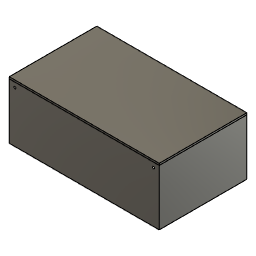
ArduinoLinInterceptor v4 (Autodesk Fusion 360 design; units mm, degrees)
Autodesk Fusion 360 part; units mm, degrees
sketch "Bottom" plane through (0, 0, 0) normal (0, 1, 0) x (1, 0, 0)
  line L0 (0, 0) -> (122, 0)
  line L1 (0, 0) -> (0, -70)
  line L2 (0, -70) -> (122, -70)
  line L3 (122, -70) -> (122, 0)
  line L4 (6, -70) -> (6, 0)
  line L5 (6, -17.75) -> (21.25, -17.75)
  line L6 (6, -66) -> (20, -66)
  line L7 (21.25, -17.75) -> (96.25, -17.75)
  line L8 (20, -66) -> (102.7, -66)
  circle A0 centre (21.25, -17.75) radius 2.5
  circle A1 centre (96.25, -17.75) radius 2.5
  circle A2 centre (20, -66) radius 2.5
  circle A3 centre (102.7, -66) radius 2.5
  point P0 (21.25, -17.75)
  point P1 (20, -66)
  dimension "d3" = 122
  dimension "d4" = 70
  dimension "d10" = 6
  dimension "d11" = 15.25
  dimension "d12" = 14
  dimension "d13" = 75
  dimension "d14" = 82.7
  dimension "d16" = 48.25
  dimension "d17" = 4
  dimension "d33" = 5
  dimension "d34" = 5
  dimension "d35" = 5
  dimension "d36" = 5
  constraint coincident L0.start L1.start
  constraint horizontal L0
  constraint perpendicular L0 L1
  constraint perpendicular L1 L2
  constraint perpendicular L2 L3
  constraint coincident L2 L4.start
  constraint coincident L0 L4.end
  constraint perpendicular L0 L4
  constraint coincident L4 L5.start
  constraint perpendicular L4 L5
  constraint coincident L4 L6.start
  constraint perpendicular L4 L6
  constraint parallel L5 L7
  constraint parallel L6 L8
  constraint coincident P0 L5.end
  constraint coincident P1 L6.end
  constraint coincident L7.end A1.centre
  constraint coincident L8.end A3.centre
  measures "d3" distance of L0.start L0.end
  measures "d4" distance of L0.start L1.end
  measures "d10" distance of L1 L4
  measures "d11" distance of L5.start P0
  measures "d12" distance of L6.start P1
  measures "d13" distance of P0 L7.end
  measures "d14" distance of P1 L8.end
  measures "d16" distance of L5 L6
  measures "d17" distance of L2 L8
  measures "d33" diameter of A0
  measures "d34" diameter of A1
  measures "d35" diameter of A2 L1
  measures "d36" diameter of A3
extrude "Extrude1" add sketch "Bottom" against normal blind 1.5 contours L0 L1 L2 L4 | L0 L2 L3 L4 | L5 L7 A0 | L5 L7 A0 | L6 L8 A2 | L6 L8 A2 | A1 | A3 makes body 1
extrude "Extrude2" add sketch "Bottom" along normal blind 45 and the other way blind 1.5 thin wall 1.5 outside contours L0 L1 L2 L4 | L0 L2 L3 L4 | L5 L7 A0 | L5 L7 A0 | L6 L8 A2 | L6 L8 A2 | A1 | A3 bodies 1
extrude "Extrude3" add sketch "Bottom" along normal blind 3.5 contours L5 L7 A0 | L5 L7 A0 | L6 L8 A2 | L6 L8 A2 | A1 | A3 bodies 1
sketch "ScrewHoles" plane through (0, 3.5, 0) normal (0, 1, 0) x (-1, 0, 0)
  circle A0 centre (-21.25, 17.75) radius 2.5
  circle A1 centre (-21.25, 17.75) radius 2.5
  circle A2 centre (-20, 66) radius 2.5
  line L0 (-21.25, 17.75) -> (-96.25, 17.75)
  circle A3 centre (-102.7, 66) radius 2.5
  line L1 (-122, 70) -> (-122, 0)
  line L2 (-6, 66) -> (-20, 66)
  line L3 (0, 0) -> (-122, 0)
  line L4 (0, 0) -> (0, 70)
  line L5 (0, 70) -> (-122, 70)
  line L6 (-6, 17.75) -> (-21.25, 17.75)
  line L7 (-6, 70) -> (-6, 0)
  line L8 (-20, 66) -> (-102.7, 66)
  circle A4 centre (-96.25, 17.75) radius 2.5
  point P0 (-20, 66)
  point P1 (-21.25, 17.75)
  dimension "d40" = 122
  dimension "d41" = 70
  dimension "d42" = 6
  dimension "d43" = 15.25
  dimension "d44" = 14
  dimension "d45" = 75
  dimension "d46" = 82.7
  dimension "d47" = 48.25
  dimension "d48" = 4
  dimension "d49" = 5
  dimension "d50" = 5
  dimension "d51" = 5
  dimension "d52" = 5
  constraint coincident L3.start L4.start
  constraint perpendicular L3 L4
  constraint perpendicular L4 L5
  constraint perpendicular L1 L5
  constraint coincident L7.start L5
  constraint coincident L7.end L3
  constraint perpendicular L3 L7
  constraint coincident L6.start L7
  constraint perpendicular L6 L7
  constraint coincident L2.start L7
  constraint perpendicular L2 L7
  constraint parallel L0 L6
  constraint parallel L2 L8
  constraint coincident P1 A0.centre
  constraint coincident P0 A2.centre
  constraint coincident L0.end A4.centre
  constraint coincident A3.centre L8.end
  measures "d40" distance of L3.start L1.end
  measures "d41" distance of L4.end L3.start
  measures "d42" distance of L4 L7
  measures "d43" distance of P1 L6.start
  measures "d44" distance of L2.start P0
  measures "d45" distance of L0.end P1
  measures "d46" distance of A3.centre P0
  measures "d47" distance of L2 L6
  measures "d48" distance of L5 L8
  measures "d49" diameter of A1
  measures "d50" diameter of A4
  measures "d51" diameter of A2
  measures "d52" diameter of A3
hole "Hole1" at (21.25, 3.5, 17.75) at (96.25, 3.5, 17.75) at (20, 3.5, 66) at (102.7, 3.5, 66) direction (0, -1, 0) diameter 1.769 depth 3.5 tip angle 118 bodies 1
thread "Thread1" "ISO Metric profile 2.0 M2x0.25 6H"
sketch "Sketch3" plane through (-1.5, 0, 0) normal (-1, 0, 0) x (0, 0, 1)
  line L0 (71.5, -1.5) -> (71.5, 45)
  line L1 (71.5, 45) -> (-1.5, 45)
  line L2 (-1.5, 45) -> (-1.5, -1.5)
  line L3 (-1.5, -1.5) -> (71.5, -1.5)
  line L4 (0, 0) -> (22.45, 0)
  line L5 (22.45, 0) -> (22.45, 3.5)
  line L6 (22.45, 3.5) -> (34.45, 3.5)
  line L7 (34.45, 3.5) -> (34.45, 15.5)
  line L8 (34.45, 15.5) -> (22.45, 15.5)
  line L9 (22.45, 15.5) -> (22.45, 3.5)
  line L10 (35, 45) -> (60, 45)
  line L11 (60, 45) -> (60, 35)
  line L12 (60, 35) -> (35, 35)
  line L13 (35, 35) -> (35, 45)
  dimension "d61" = 22.45
  dimension "d62" = 3.5
  dimension "d63" = 12
  dimension "d64" = 12
  dimension "d70" = 25
  dimension "d71" = 10
  dimension "d72" = 11.5
  constraint coincident L4.start origin
  constraint perpendicular L2 L4
  constraint perpendicular L4 L5
  constraint horizontal L6
  constraint vertical L7
  constraint horizontal L8
  constraint vertical L9
  constraint horizontal L10
  constraint vertical L11
  constraint horizontal L12
  constraint vertical L13
  constraint coincident L1 L10.start
  measures "d61" distance of L4.start L4.end
  measures "d62" distance of L4.end L5.end
  measures "d63" distance of L5.end L6.end
  measures "d64" distance of L5.end L8.end
  measures "d70" distance of L10.start L10.end
  measures "d71" distance of L10.start L12.end
  measures "d72" distance of L0 L11
extrude "Extrude4" cut sketch "Sketch3" against normal blind 1.5 contours L1 L10 L11 L12 L13 | L6 L7 L8 L9 bodies 1
sketch "Sketch4" plane through (0, 0, -1.5) normal (0, 0, -1) x (-1, 0, 0)
  line L0 (1.5, -1.5) -> (1.5, 45)
  line L1 (1.5, 45) -> (-123.5, 45)
  line L2 (-123.5, 45) -> (-123.5, -1.5)
  line L3 (-123.5, -1.5) -> (1.5, -1.5)
  line L4 (-83.5, 45) -> (-58.5, 45)
  line L5 (-58.5, 45) -> (-58.5, 35)
  line L6 (-58.5, 35) -> (-83.5, 35)
  line L7 (-83.5, 35) -> (-83.5, 45)
  line L8 (-122.2473, 45) -> (-122.2473, -1.5)
  dimension "d74" = 25
  dimension "d75" = 10
  dimension "d76" = 60
  constraint horizontal L4
  constraint vertical L5
  constraint horizontal L6
  constraint vertical L7
  constraint coincident L1 L4.start
  constraint coincident L1 L8.start
  constraint coincident L3 L8.end
  constraint perpendicular L3 L8
  measures "d74" distance of L4.start L4.end
  measures "d75" distance of L4.start L6.end
  measures "d76" distance of L0 L5
extrude "Extrude5" [suppressed]
sketch "Top" plane through (0, 45, 0) normal (0, 1, 0) x (-1, 0, 0)
  line L0 (0, 0) -> (-122, 0)
  line L1 (-122, 0) -> (-122, 70)
  line L2 (-122, 70) -> (0, 70)
  line L3 (0, 35) -> (0, 0)
  line L4 (0, 60) -> (1.5, 60)
  line L5 (1.5, 60) -> (1.5, 71.5)
  line L6 (1.5, 71.5) -> (-123.5, 71.5)
  line L7 (-123.5, 71.5) -> (-123.5, -1.5)
  line L8 (-123.5, -1.5) -> (1.5, -1.5)
  line L9 (0, 0) -> (-122, 0)
  line L10 (-122, 0) -> (-122, 70)
  line L11 (-122, 70) -> (0, 70)
  line L12 (0, 70) -> (0, 0)
  line L13 (1.5, 35) -> (0, 35)
  line L14 (1.5, -1.5) -> (1.5, 35)
  line L15 (0, 70) -> (0, 60)
  constraint horizontal L9
  constraint vertical L10
  constraint horizontal L11
  constraint vertical L12
  constraint coincident L1.end L2.start
  constraint coincident L0.start L3.end
extrude "Extrude6" add sketch "Top" along normal blind 1.5 separate body contours L0 L1 L2 L3 L9 L10 L11 L12 L15 makes body 2
extrude "Extrude7" add sketch "Top" along normal blind 1.5 thin wall 1.5 outside contours L0 L1 L2 L3 L9 L10 L11 L12 L15 bodies 2
extrude "Extrude8" add sketch "Top" against normal blind 1 contours L0 L1 L2 L3 L9 L10 L11 L12 L15 bodies 2
extrude "Extrude9" cut sketch "Top" against normal blind 1 thin wall 0.25 inside contours L0 L1 L2 L3 L9 L10 L11 L12 L15 bodies 2
sketch "Sketch6" plane through (0, 45, 0) normal (0, -1, 0) x (1, 0, 0)
  line L0 (121.75, 69.75) -> (121.75, 0.25)
  line L1 (121.75, 0.25) -> (0.25, 0.25)
  line L2 (0.25, 0.25) -> (0.25, 69.75)
  line L3 (0.25, 69.75) -> (121.75, 69.75)
  line L4 (123.5, 71.5) -> (-1.5, 71.5)
  line L5 (-1.5, 71.5) -> (-1.5, -1.5)
  line L6 (-1.5, -1.5) -> (123.5, -1.5)
  line L7 (123.5, -1.5) -> (123.5, 71.5)
sketch "Sketch7" plane through (0, 44, 0) normal (0, -1, 0) x (1, 0, 0)
  line L0 (121.75, 0.25) -> (121.75, 69.75)
  line L1 (121.75, 69.75) -> (0.25, 69.75)
  line L2 (0.25, 69.75) -> (0.25, 0.25)
  line L3 (0.25, 0.25) -> (121.75, 0.25)
  line L4 (0.25, 67.75) -> (121.75, 67.75)
  line L5 (0.25, 2.25) -> (121.75, 2.25)
  line L6 (115.75, 69.75) -> (115.75, 0.25)
  line L7 (6.25, 69.75) -> (6.25, 0.25)
  dimension "d93" = 6
  dimension "d94" = 6
  dimension "d95" = 2
  dimension "d96" = 2
  constraint coincident L2 L4.start
  constraint coincident L0 L4.end
  constraint perpendicular L0 L4
  constraint coincident L2 L5.start
  constraint coincident L0 L5.end
  constraint perpendicular L0 L5
  constraint coincident L1 L6.start
  constraint coincident L3 L6.end
  constraint perpendicular L3 L6
  constraint coincident L1 L7.start
  constraint coincident L3 L7.end
  constraint perpendicular L3 L7
  measures "d93" distance of L2 L7
  measures "d94" distance of L0 L6
  measures "d95" distance of L1 L4
  measures "d96" distance of L3 L5
extrude "Extrude10" add sketch "Sketch7" along normal blind 6 contours L0 L3 L5 L6 | L0 L1 L4 L6 | L2 L3 L5 L7 | L1 L2 L4 L7 bodies 2
sketch "Sketch8" plane through (0, 0, 69.75) normal (0, 0, 1) x (1, 0, 0)
  line L0 (121.75, 45) -> (0.25, 45)
  line L1 (0.25, 45) -> (0.25, 38)
  line L2 (0.25, 38) -> (6.25, 38)
  line L3 (6.25, 38) -> (6.25, 44)
  line L4 (6.25, 44) -> (115.75, 44)
  line L5 (115.75, 44) -> (115.75, 38)
  line L6 (115.75, 38) -> (121.75, 38)
  line L7 (121.75, 38) -> (121.75, 45)
  line L8 (115.75, 41) -> (121.75, 41)
  line L9 (6.25, 41) -> (0.25, 41)
  point P0 (0, 61)
  point P1 (3.25, 41)
  point P2 (118.75, 41)
  constraint midpoint L5 L8.start
  constraint coincident L7 L8.end
  constraint perpendicular L7 L8
  constraint midpoint L8 P2
  constraint midpoint L3 L9.start
  constraint coincident L1 L9.end
  constraint perpendicular L1 L9
  constraint midpoint P1 L9
sketch "Sketch9" plane through (0, 0, 0.25) normal (0, 0, -1) x (-1, 0, 0)
  line L0 (-0.25, 45) -> (-121.75, 45)
  line L1 (-121.75, 45) -> (-121.75, 38)
  line L2 (-121.75, 38) -> (-115.75, 38)
  line L3 (-115.75, 38) -> (-115.75, 44)
  line L4 (-115.75, 44) -> (-6.25, 44)
  line L5 (-6.25, 44) -> (-6.25, 38)
  line L6 (-6.25, 38) -> (-0.25, 38)
  line L7 (-0.25, 38) -> (-0.25, 45)
  line L8 (-0.25, 45) -> (-0.25, 38)
  line L9 (-0.25, 38) -> (-6.25, 38)
  line L10 (-115.75, 44) -> (-115.75, 38)
  line L11 (-6.25, 44) -> (-115.75, 44)
  line L12 (-6.25, 38) -> (-6.25, 44)
  line L13 (-115.75, 38) -> (-121.75, 38)
  line L14 (-121.75, 38) -> (-121.75, 45)
  line L15 (-121.75, 45) -> (-0.25, 45)
  line L16 (-115.75, 41) -> (-121.75, 41)
  line L17 (-6.25, 41) -> (-0.25, 41)
  point P0 (-118.75, 41)
  point P1 (-3.25, 41)
  dimension "d105" = 7
  constraint midpoint L16.start L10
  constraint coincident L16.end L14
  constraint perpendicular L14 L16
  constraint midpoint P0 L16
  constraint midpoint L5 L17.start
  constraint coincident L8 L17.end
  constraint perpendicular L8 L17
  constraint midpoint P1 L17
  measures "d105" distance of L0.start L6.end
hole "Hole2" at (3.25, 41, 69.75) at (118.75, 41, 69.75) direction (0, 0, -1) diameter 1.769 depth 2 tip angle 180 bodies 2
thread "Thread2" "ISO Metric profile 2.0 M2x0.25 6H" major diameter 2.0555 minor diameter 1.7694 pitch 0.25 angle 60 resizes the face on face at (119.2112, 41.7547, 69.0833) on face at (2.6815, 40.3224, 69.0833) on bodies 2
hole "Hole3" at (118.75, 41, 0.25) at (3.25, 41, 0.25) direction (0, 0, 1) diameter 1.769 depth 2 tip angle 180 bodies 2
thread "Thread3" "ISO Metric profile 2.0 M2x0.25 6H" major diameter 2.0555 minor diameter 1.7694 pitch 0.25 angle 60 resizes the face on face at (2.6815, 41.6776, 0.9167) on face at (119.2112, 40.2453, 0.9167) on bodies 2
sketch "Sketch10" plane through (0, 0, -1.5) normal (0, 0, -1) x (-1, 0, 0)
  line L0 (1.5, -1.5) -> (1.5, 45)
  line L1 (1.5, 45) -> (-123.5, 45)
  line L2 (-123.5, 45) -> (-123.5, -1.5)
  line L3 (-123.5, -1.5) -> (1.5, -1.5)
  line L4 (-123.5, 44) -> (-115.75, 44)
  line L5 (-115.75, 44) -> (-115.75, 38)
  line L6 (-115.75, 38) -> (-121.75, 38)
  line L7 (-121.75, 38) -> (-121.75, 44)
  line L8 (-121.75, 41) -> (-115.75, 41)
  line L9 (-61, 45) -> (-61, -1.5)
  line L10 (1.5, 44) -> (-6.25, 44)
  line L11 (-6.25, 38) -> (-0.25, 38)
  line L12 (-6.25, 44) -> (-6.25, 38)
  line L13 (-0.25, 38) -> (-0.25, 44)
  line L14 (-0.25, 41) -> (-6.25, 41)
  point P0 (-118.75, 41)
  point P1 (-3.25, 41)
  dimension "d112" = 7.75
  dimension "d113" = 1
  dimension "d114" = 6
  dimension "d115" = 6
  constraint coincident L2 L4.start
  constraint perpendicular L4 L5
  constraint perpendicular L5 L6
  constraint coincident L4 L7.end
  constraint perpendicular L4 L7
  constraint midpoint L7 L8.start
  constraint midpoint L5 L8.end
  constraint midpoint L8 P0
  constraint midpoint L1 L9.start
  constraint midpoint L3 L9.end
  constraint symmetric L4.start L9 L10.start
  constraint symmetric L4.end L9 L10.end
  constraint symmetric L5.end L9 L11.start
  constraint symmetric L6.end L9 L11.end
  constraint symmetric L7.end L9 L13.end
  constraint symmetric L8.start L9 L14.start
  constraint symmetric L8.end L9 L14.end
  constraint symmetric P0 L9 P1
  measures "d112" distance of L4.start L4.end
  measures "d113" distance of L1 L4
  measures "d114" distance of L5 L7
  measures "d115" distance of L4 L6
sketch "Sketch11" plane through (0, 0, 71.5) normal (0, 0, 1) x (1, 0, 0)
  line L0 (123.5, -1.5) -> (123.5, 45)
  line L1 (123.5, 45) -> (-1.5, 45)
  line L2 (-1.5, 45) -> (-1.5, -1.5)
  line L3 (-1.5, -1.5) -> (123.5, -1.5)
  line L4 (0, 45) -> (0, 0)
  line L5 (0.25, 41) -> (6.25, 41)
  line L6 (123.5, -1.5) -> (-1.5, -1.5)
  line L7 (123.5, 45) -> (123.5, -1.5)
  line L8 (-1.5, -1.5) -> (-1.5, 45)
  line L9 (121.75, 41) -> (115.75, 41)
  line L10 (0.25, 38) -> (0.25, 44)
  line L11 (123.5, 44) -> (115.75, 44)
  line L12 (6.25, 38) -> (0.25, 38)
  line L13 (115.75, 44) -> (115.75, 38)
  line L14 (61, 45) -> (61, -1.5)
  line L15 (-1.5, 45) -> (123.5, 45)
  line L16 (115.75, 38) -> (121.75, 38)
  line L17 (121.75, 38) -> (121.75, 44)
  line L18 (-1.5, 44) -> (6.25, 44)
  line L19 (6.25, 44) -> (6.25, 38)
  point P0 (3.25, 41)
  point P1 (118.75, 41)
  dimension "d116" = 7.75
  dimension "d117" = 1
  dimension "d118" = 6
  dimension "d119" = 6
  constraint coincident L1 L4.start
  constraint coincident L4.end origin
  constraint perpendicular L1 L4
  constraint coincident L11.start L7
  constraint perpendicular L11 L13
  constraint perpendicular L13 L16
  constraint coincident L17.end L11
  constraint perpendicular L11 L17
  constraint midpoint L9.start L17
  constraint midpoint L9.end L13
  constraint midpoint P1 L9
  constraint midpoint L14.start L15
  constraint midpoint L14.end L6
  constraint symmetric L11.start L18.start L14
  constraint symmetric L11.end L18.end L14
  constraint symmetric L12.start L13.end L14
  constraint symmetric L10.start L16.end L14
  constraint symmetric L17.end L10.end L14
  constraint symmetric L9.start L5.start L14
  constraint symmetric L9.end L5.end L14
  constraint symmetric P0 P1 L14
  measures "d116" distance of L11.start L11.end
  measures "d117" distance of L11 L15
  measures "d118" distance of L13 L17
  measures "d119" distance of L11 L16
hole "Hole4" at (118.75, 41, 71.5) at (3.25, 41, 71.5) direction (0, 0, -1) diameter 1.769 depth 1.5 tip angle 180 bodies 1
thread "Thread4" "ISO Metric profile 2.0 M2x0.25 6H" major diameter 2.0555 minor diameter 1.7694 pitch 0.25 angle 60 resizes the face on face at (2.7159, 40.2949, 71) on face at (119.2112, 41.7547, 71) on bodies 1
hole "Hole5" at (118.75, 41, -1.5) at (3.25, 41, -1.5) direction (0, 0, 1) diameter 1.769 depth 1.5 tip angle 180 bodies 1
thread "Thread5" "ISO Metric profile 2.0 M2x0.25 6H" major diameter 2.0555 minor diameter 1.7694 pitch 0.25 angle 60 resizes the face on face at (119.173, 40.2232, -1) on face at (2.7159, 41.7051, -1) on bodies 1
equation "BottomLength = 122 mm"
equation "BottomWidth = 70 mm"
equation "d3 = BottomLength"
equation "d4 = BottomWidth"
equation "DistScrewsLeft = 82.7 mm"
equation "DistScrewsRight = 75 mm"
equation "ScrewToSideRight = 15.25 mm"
equation "ScrewToSideLeft = 14 mm"
equation "DistPortSideToBoard = 6 mm"
equation "d10 = DistPortSideToBoard"
equation "d11 = ScrewToSideRight"
equation "d12 = ScrewToSideLeft"
equation "d13 = DistScrewsRight"
equation "d14 = DistScrewsLeft"
equation "DistScrewSides = 48.25 mm"
equation "d16 = DistScrewSides"
equation "d17 = ScrewCenterToLeftSide"
equation "ScrewCenterToLeftSide = 4 mm"
equation "Wall = 1.5 mm"
equation "d20 = -Wall"
equation "d22 = Wall"
equation "d23 = Height"
equation "d25 = Wall"
equation "d26 = Wall"
equation "Height = 45 mm"
equation "RightSideToUSB = 7 mm"
equation "USBWidth = 12 mm"
equation "BottomToBoard = 3.5 mm"
equation "ScrewCylDiameter = 5 mm"
equation "d33 = ScrewCylDiameter"
equation "d34 = ScrewCylDiameter"
equation "d35 = ScrewCylDiameter"
equation "d36 = ScrewCylDiameter"
equation "d37 = BottomToBoard"
equation "d40 = BottomLength"
equation "d41 = BottomWidth"
equation "d42 = DistPortSideToBoard"
equation "d43 = ScrewToSideRight"
equation "d44 = ScrewToSideLeft"
equation "d45 = DistScrewsRight"
equation "d46 = DistScrewsLeft"
equation "d47 = DistScrewSides"
equation "d48 = ScrewCenterToLeftSide"
equation "d49 = ScrewCylDiameter"
equation "d50 = ScrewCylDiameter"
equation "d51 = ScrewCylDiameter"
equation "d52 = ScrewCylDiameter"
equation "d53 = BottomToBoard"
equation "BoardThickness = 1.5 mm"
equation "USBHeight = 12 mm"
equation "RightWallToUSB = BottomWidth - ( DistScrewSides + ScrewCenterToLeftSide + BoardSideToScrewCenter ) + RightSideToUSB"
equation "BoardSideToScrewCenter = 2.3 mm"
equation "RightBoardSideToUSB = RightSideToUSB - BoardSideToScrewCenter"
equation "d61 = RightWallToUSB"
equation "d62 = BottomToBoard"
equation "d63 = USBWidth"
equation "d64 = USBHeight"
equation "d65 = -Wall"
equation "CableHoleWidth = 25 mm"
equation "CableHoleHeight = 10 mm"
equation "LeftWallToCableHole = 10 mm"
equation "d70 = CableHoleWidth"
equation "d71 = CableHoleHeight"
equation "d72 = LeftWallToCableHole + Wall"
equation "PortSideToCableHole = 60 mm"
equation "d74 = CableHoleWidth"
equation "d75 = CableHoleHeight"
equation "d76 = PortSideToCableHole"
equation "d77 = -Wall"
equation "d79 = Wall"
equation "d81 = Wall"
equation "d82 = Wall"
equation "d84 = -LidOffset"
equation "d86 = SpacingBetweenInterlockingComponents"
equation "d87 = -LidOffset"
equation "SpacingBetweenInterlockingComponents = 0.25 mm"
equation "ScrewTabDepth = 2 mm"
equation "ScrewTabWidth = 6 mm"
equation "ScrewTabHeight = 6 mm"
equation "d93 = ScrewTabWidth"
equation "d94 = ScrewTabWidth"
equation "d95 = ScrewTabDepth"
equation "d96 = ScrewTabDepth"
equation "d97 = ScrewTabHeight"
equation "d99 = ScrewTabDepth"
equation "d102 = ScrewTabDepth"
equation "LidOffset = 1 mm"
equation "d112 = Wall + SpacingBetweenInterlockingComponents + ScrewTabWidth"
equation "d113 = LidOffset"
equation "d114 = ScrewTabWidth"
equation "d115 = ScrewTabHeight"
equation "d116 = Wall + SpacingBetweenInterlockingComponents + ScrewTabWidth"
equation "d117 = LidOffset"
equation "d118 = ScrewTabWidth"
equation "d119 = ScrewTabHeight"
equation "d120 = Wall"
equation "d123 = Wall"
